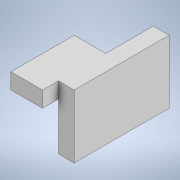
# Autodesk Inventor part: wobble goal arm
Saved by Autodesk Inventor 2020.1 (Build 241239000, 239)
## iProperties
Created: 2020-09-26
Part Number: wobble goal arm
Material: Generic
Document SubType Name: Modeling
Designer: elois
Density: 1 g/cm^3
Appearance: Default
Author: elois
Autodesk Inventor part; units mm, degrees
ref_plane "YZ Plane" through (0, 0, 0) normal (1, 0, 0) x (0, 1, 0)
ref_plane "XZ Plane" through (0, 0, 0) normal (0, 1, 0) x (-1, 0, 0)
ref_plane "XY Plane" through (0, 0, 0) normal (0, 0, 1) x (1, 0, 0)
sketch "Sketch1" plane through (0, 0, 0) normal (0, 1, 0) x (-1, 0, 0)
  line L0 (0, 0) -> (50.8, 0)
  line L1 (50.8, 0) -> (50.8, -25.4)
  line L2 (50.8, -25.4) -> (0, -25.4)
  line L3 (0, -25.4) -> (0, 0)
  dimension "d0" = 50.8
  dimension "d1" = 25.4
  dimension "d2" = 50.8
  dimension "d3" = 90
  constraints: 8 end point, 2 perpendicular, 1 horizontal
  measures "d0" distance of L0.start L0.end
  measures "d1" distance of L0.end L1.end
  measures "d2" distance of L1.end L2.end
  measures "d3" angle of L1 L2
extrude "Extrusion1" add sketch "Sketch1" along normal blind 12.7
sketch "Sketch2" plane through (0, 0, -25.4) normal (0, 0, -1) x (-1, 0, 0)
  line L0 (0, 12.7) -> (50.8, 12.7) projected
  line L1 (50.8, 12.7) -> (12.7, 12.7)
  line L2 (12.7, 12.7) -> (12.7, -76.2)
  line L3 (12.7, 12.7) -> (88.9, 12.7)
  line L4 (88.9, 12.7) -> (88.9, -38.1)
  line L5 (88.9, -38.1) -> (12.7, -38.1)
  line L6 (12.7, -38.1) -> (12.7, 12.7)
  point P0 (0, 0)
  point P1 (12.7, -38.1)
  dimension "d11" = 76.2
  dimension "d12" = 50.8
  constraints: 12 end point, 2 parallel, 1 horizontal, 1 perpendicular, 1 point on line
  measures "d11" distance of L4.end L5.end
  measures "d12" distance of L3.end L4.end
extrude "Extrusion2" add sketch "Sketch2" along normal blind 12.7
move or copy body "Move Body1" bodies to move or copy 1 copy no rotation origin (0, 0, 0) rotation axis (0, 1, 0) rotation angle -90 translate (-76.2, 0, 25.4)
body "Solid1"
